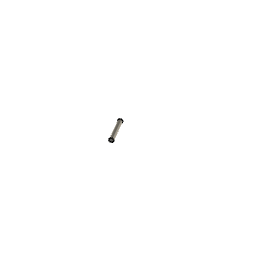
Tripod4 v1 (Autodesk Fusion 360 design; units mm, degrees)
Autodesk Fusion 360 part; units mm, degrees
sketch "Sketch1" plane through (5, -8.6603, 0) normal (0.5, -0.866025, 0) x (0.866025, 0.5, 0)
  arc A0 (-70.01, 5) -> (-65.01, 0) centre (-65.01, 5) ccw
  line L0 (-65.01, 0) -> (-50.01, 0)
  line L1 (-50.01, 0) -> (-50.01, 18.5)
  line L2 (-50.01, 18.5) -> (-70.01, 18.5)
  line L3 (-70.01, 18.5) -> (-70.01, 5)
  circle A1 centre (-60.01, 8) radius 1.6
  circle A2 centre (-60.01, 8) radius 1.5
  dimension "d57" = 3
  constraint concentric A1 A2
  measures "d57" diameter of A2
extrude "Extrude1" add sketch "Sketch1" against normal blind 20 contours A2
